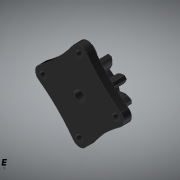
# Autodesk Inventor part: m2z10
Saved by Autodesk Inventor 2020 (Build 240168000, 168)
## iProperties
Created: 2019-05-28
Part Number: m2z10
Material: アルミニウム 2014-T4
Document SubType Name: Modeling
Designer: hamaa
Density: 2.8 g/cm^3
Appearance: サテン
Mass: 8.90635 g
Surface Area: 23.1017 cm^2
Volume: 3.18084 cm^3
Author: hamaa
Autodesk Inventor part; units mm, degrees
note: some values were not read from the file. Chosen so that the rebuilt part matches the saved one: sketch regions of "押し出し5".
ref_plane "YZ Plane" through (0, 0, 0) normal (1, 0, 0) x (0, 1, 0)
ref_plane "XZ Plane" through (0, 0, 0) normal (0, 1, 0) x (-1, 0, 0)
ref_plane "XY Plane" through (0, 0, 0) normal (0, 0, 1) x (1, 0, 0)
sketch "スケッチ1" plane through (0, 0, 0) normal (0, 0, 1) x (1, 0, 0)
  arc A0 (149.895, 114.5174) -> (149.8316, 114.302) centre (151.0075, 114.073) ccw
  arc A1 (150.3048, 115.256) -> (149.895, 114.5174) centre (153.0017, 113.2765) ccw
  arc A2 (151.645, 116.5804) -> (150.3048, 115.256) centre (155.1281, 111.7157) ccw
  arc A3 (144.0343, 113.5196) -> (144.1097, 113.3081) centre (145.1956, 113.8141) ccw
  arc A4 (143.9318, 114.3581) -> (144.0343, 113.5196) centre (147.2771, 114.3418) ccw
  arc A5 (144.2375, 116.2174) -> (143.9318, 114.3581) centre (149.9148, 114.329) ccw
  arc A6 (139.8794, 109.2677) -> (140.0647, 109.1408) centre (140.6459, 110.1884) ccw
  arc A7 (139.3036, 109.8857) -> (139.8794, 109.2677) centre (142.0196, 111.8388) ccw
  arc A8 (138.4581, 111.5696) -> (139.3036, 109.8857) centre (144.1611, 113.3789) ccw
  arc A9 (139.0173, 103.3856) -> (139.2417, 103.3918) centre (139.0961, 104.581) ccw
  arc A10 (138.1882, 103.5471) -> (139.0173, 103.3856) centre (139.2374, 106.7236) ccw
  arc A11 (136.5144, 104.4124) -> (138.1882, 103.5471) centre (140.0647, 109.2283) ccw
  arc A12 (141.7772, 98.1201) -> (141.9551, 98.2571) centre (141.1383, 99.1335) ccw
  arc A13 (141.0115, 97.7634) -> (141.7772, 98.1201) centre (139.9932, 100.95) ccw
  arc A14 (139.1487, 97.4797) -> (141.0115, 97.7634) centre (139.1903, 103.4626) ccw
  arc A15 (147.105, 95.4824) -> (147.1684, 95.6978) centre (145.9925, 95.9268) ccw
  arc A16 (146.6952, 94.7438) -> (147.105, 95.4824) centre (143.9983, 96.7233) ccw
  arc A17 (145.355, 93.4194) -> (146.6952, 94.7438) centre (141.8719, 98.2841) ccw
  arc A18 (152.9656, 96.4802) -> (152.8903, 96.6917) centre (151.8044, 96.1857) ccw
  arc A19 (153.0682, 95.6417) -> (152.9656, 96.4802) centre (149.7229, 95.658) ccw
  arc A20 (152.7625, 93.7824) -> (153.0682, 95.6417) centre (147.0852, 95.6708) ccw
  arc A21 (157.1206, 100.7321) -> (156.9353, 100.859) centre (156.3541, 99.8114) ccw
  arc A22 (157.6964, 100.1141) -> (157.1206, 100.7321) centre (154.9804, 98.161) ccw
  arc A23 (158.5419, 98.4302) -> (157.6964, 100.1141) centre (152.8389, 96.6209) ccw
  arc A24 (157.9827, 106.6143) -> (157.7583, 106.608) centre (157.9039, 105.4188) ccw
  arc A25 (158.8118, 106.4527) -> (157.9827, 106.6143) centre (157.7626, 103.2762) ccw
  arc A26 (160.4856, 105.5874) -> (158.8118, 106.4527) centre (156.9353, 100.7715) ccw
  arc A27 (155.2228, 111.8797) -> (155.0449, 111.7427) centre (155.8617, 110.8663) ccw
  arc A28 (155.9885, 112.2364) -> (155.2228, 111.8797) centre (157.0068, 109.0498) ccw
  arc A29 (157.8512, 112.5201) -> (155.9885, 112.2364) centre (157.8097, 106.5372) ccw
  arc A30 (147.1684, 114.302) -> (147.105, 114.5174) centre (145.9925, 114.073) ccw
  arc A31 (147.105, 114.5174) -> (146.6952, 115.256) centre (143.9983, 113.2765) ccw
  arc A32 (146.6952, 115.256) -> (145.355, 116.5804) centre (141.8719, 111.7157) ccw
  arc A33 (141.9551, 111.7427) -> (141.7772, 111.8797) centre (141.1383, 110.8663) ccw
  arc A34 (141.7772, 111.8797) -> (141.0115, 112.2364) centre (139.9932, 109.0498) ccw
  arc A35 (141.0115, 112.2364) -> (139.1487, 112.5201) centre (139.1903, 106.5372) ccw
  arc A36 (139.2417, 106.608) -> (139.0173, 106.6143) centre (139.0961, 105.4188) ccw
  arc A37 (139.0173, 106.6143) -> (138.1882, 106.4527) centre (139.2374, 103.2762) ccw
  arc A38 (138.1882, 106.4527) -> (136.5144, 105.5874) centre (140.0647, 100.7715) ccw
  arc A39 (140.0647, 100.859) -> (139.8794, 100.7321) centre (140.6459, 99.8114) ccw
  arc A40 (139.8794, 100.7321) -> (139.3036, 100.1141) centre (142.0196, 98.161) ccw
  arc A41 (139.3036, 100.1141) -> (138.4581, 98.4302) centre (144.1611, 96.6209) ccw
  arc A42 (144.1097, 96.6917) -> (144.0343, 96.4802) centre (145.1956, 96.1857) ccw
  arc A43 (144.0343, 96.4802) -> (143.9318, 95.6417) centre (147.2771, 95.658) ccw
  arc A44 (143.9318, 95.6417) -> (144.2375, 93.7824) centre (149.9148, 95.6708) ccw
  arc A45 (149.8316, 95.6978) -> (149.895, 95.4824) centre (151.0075, 95.9268) ccw
  arc A46 (149.895, 95.4824) -> (150.3048, 94.7438) centre (153.0017, 96.7233) ccw
  arc A47 (150.3048, 94.7438) -> (151.645, 93.4194) centre (155.1281, 98.2841) ccw
  arc A48 (155.0449, 98.2571) -> (155.2228, 98.1201) centre (155.8617, 99.1335) ccw
  arc A49 (155.2228, 98.1201) -> (155.9885, 97.7634) centre (157.0068, 100.95) ccw
  arc A50 (155.9885, 97.7634) -> (157.8512, 97.4797) centre (157.8097, 103.4626) ccw
  arc A51 (157.7583, 103.3918) -> (157.9827, 103.3856) centre (157.9039, 104.581) ccw
  arc A52 (157.9827, 103.3856) -> (158.8118, 103.5471) centre (157.7626, 106.7236) ccw
  arc A53 (158.8118, 103.5471) -> (160.4856, 104.4124) centre (156.9353, 109.2283) ccw
  arc A54 (156.9353, 109.1408) -> (157.1206, 109.2677) centre (156.3541, 110.1884) ccw
  arc A55 (157.1206, 109.2677) -> (157.6964, 109.8857) centre (154.9804, 111.8388) ccw
  arc A56 (157.6964, 109.8857) -> (158.5419, 111.5696) centre (152.8389, 113.3789) ccw
  arc A57 (152.8903, 113.3081) -> (152.9656, 113.5196) centre (151.8044, 113.8141) ccw
  arc A58 (152.9656, 113.5196) -> (153.0682, 114.3581) centre (149.7229, 114.3418) ccw
  arc A59 (153.0682, 114.3581) -> (152.7625, 116.2174) centre (147.0852, 114.329) ccw
  arc A60 (149.5628, 112.4242) -> (147.4372, 112.4242) centre (148.5, 104.9999) ccw
  arc A61 (144.9959, 111.631) -> (143.2763, 110.3816) centre (148.5, 104.9999) ccw
  arc A62 (141.7675, 108.3049) -> (141.1106, 106.2833) centre (148.5, 104.9999) ccw
  arc A63 (141.1106, 103.7165) -> (141.7675, 101.6949) centre (148.5, 104.9999) ccw
  arc A64 (143.2763, 99.6182) -> (144.9959, 98.3688) centre (148.5, 104.9999) ccw
  arc A65 (147.4372, 97.5756) -> (149.5628, 97.5756) centre (148.5, 104.9999) ccw
  arc A66 (152.0041, 98.3688) -> (153.7237, 99.6182) centre (148.5, 104.9999) ccw
  arc A67 (155.2325, 101.6949) -> (155.8894, 103.7165) centre (148.5, 104.9999) ccw
  arc A68 (155.8894, 106.2833) -> (155.2325, 108.3049) centre (148.5, 104.9999) ccw
  arc A69 (153.7237, 110.3816) -> (152.0041, 111.631) centre (148.5, 104.9999) ccw
  arc A70 (145.355, 116.5804) -> (144.2375, 116.2174) centre (148.5, 104.9999) ccw
  arc A71 (139.1487, 112.5201) -> (138.4581, 111.5696) centre (148.5, 104.9999) ccw
  arc A72 (136.5144, 105.5874) -> (136.5144, 104.4124) centre (148.5, 104.9999) ccw
  arc A73 (138.4581, 98.4302) -> (139.1487, 97.4797) centre (148.5, 104.9999) ccw
  arc A74 (144.2375, 93.7824) -> (145.355, 93.4194) centre (148.5, 104.9999) ccw
  arc A75 (151.645, 93.4194) -> (152.7625, 93.7824) centre (148.5, 104.9999) ccw
  arc A76 (157.8512, 97.4797) -> (158.5419, 98.4302) centre (148.5, 104.9999) ccw
  arc A77 (160.4856, 104.4124) -> (160.4856, 105.5874) centre (148.5, 104.9999) ccw
  arc A78 (158.5419, 111.5696) -> (157.8512, 112.5201) centre (148.5, 104.9999) ccw
  arc A79 (152.7625, 116.2174) -> (151.645, 116.5804) centre (148.5, 104.9999) ccw
  line L0 (149.5628, 112.4242) -> (149.8316, 114.302)
  line L1 (144.9959, 111.631) -> (144.1097, 113.3081)
  line L2 (141.7675, 108.3049) -> (140.0647, 109.1408)
  line L3 (141.1106, 103.7165) -> (139.2417, 103.3918)
  line L4 (143.2763, 99.6182) -> (141.9551, 98.2571)
  line L5 (147.4372, 97.5756) -> (147.1684, 95.6978)
  line L6 (152.0041, 98.3688) -> (152.8903, 96.6917)
  line L7 (155.2325, 101.6949) -> (156.9353, 100.859)
  line L8 (155.8894, 106.2833) -> (157.7583, 106.608)
  line L9 (153.7237, 110.3816) -> (155.0449, 111.7427)
  line L10 (147.4372, 112.4242) -> (147.1684, 114.302)
  line L11 (143.2763, 110.3816) -> (141.9551, 111.7427)
  line L12 (141.1106, 106.2833) -> (139.2417, 106.608)
  line L13 (141.7675, 101.6949) -> (140.0647, 100.859)
  line L14 (144.9959, 98.3688) -> (144.1097, 96.6917)
  line L15 (149.5628, 97.5756) -> (149.8316, 95.6978)
  line L16 (153.7237, 99.6182) -> (155.0449, 98.2571)
  line L17 (155.8894, 103.7165) -> (157.7583, 103.3918)
  line L18 (155.2325, 108.3049) -> (156.9353, 109.1408)
  line L19 (152.0041, 111.631) -> (152.8903, 113.3081)
  line L20 (134.5, 105) -> (162.5, 105)
  line L21 (148.5, 91) -> (148.5, 119)
  line L22 (180.5, 116.9999) -> (250.5, 116.9999)
  line L23 (180.5, 108.9999) -> (250.5, 108.9999)
  line L24 (180.5, 100.9999) -> (250.5, 100.9999)
  line L25 (180.5, 92.9999) -> (250.5, 92.9999)
  line L26 (180.5, 84.9999) -> (250.5, 84.9999)
  line L27 (180.5, 76.9999) -> (250.5, 76.9999)
  line L28 (180.5, 68.9999) -> (250.5, 68.9999)
  line L29 (180.5, 60.9999) -> (250.5, 60.9999)
  line L30 (180.5, 52.9999) -> (250.5, 52.9999)
  line L31 (180.5, 44.9999) -> (250.5, 44.9999)
  line L32 (180.5, 36.9999) -> (250.5, 36.9999)
  line L33 (180.5, 28.9999) -> (250.5, 28.9999)
  line L34 (180.5, 20.9999) -> (250.5, 20.9999)
  line L35 (180.5, 116.9999) -> (180.5, 20.9999)
  line L36 (250.5, 116.9999) -> (250.5, 20.9999)
  line L37 (215.5, 108.9999) -> (215.5, 20.9999)
  point P0 (0, 0)
  point P1 (186.5, 111)
  point P2 (189, 103)
  point P3 (189, 95)
  point P4 (186.5, 87)
  point P5 (189, 79)
  point P6 (184, 71)
  point P7 (186.5, 63)
  point P8 (186.5, 55)
  point P9 (186.5, 47)
  point P10 (189, 39)
  point P11 (189, 31)
  point P12 (186.5, 23)
  point P13 (216.5, 103)
  point P14 (231.5, 95)
  point P15 (232.75, 87)
  point P16 (229, 79)
  point P17 (231.5, 71)
  point P18 (225.25, 63)
  point P19 (231.5, 55)
  point P20 (231.5, 47)
  point P21 (226.5, 39)
  point P22 (234, 31)
  point P23 (234, 23)
  point P24 (149.5, 132.5)
  point P25 (149.5, 126.5)
  point P26 (166.75, 132.5)
  point P27 (167.8125, 126.5)
  constraints: 160 point on circle, 80 centre point, 72 end point, 60 tangent, 57 equal radius, 23 parallel, 2 horizontal, 2 midpoint, 2 perpendicular, 55 other
extrude "押し出し1" add sketch "スケッチ1" along normal blind 5 contours A1 A2 A79 A59 A58 A57 L19 A69 L9 A27 A28 A29 A78 A56 A55 A54 L18 A68 L8 A24 A25 A26 A77 L20 L21 A60 L0 A0 | L21 L20 A72 A38 A37 A36 L12 A62 L2 A6 A7 A8 A71 A35 A34 A33 L11 A61 L1 A3 A4 A5 A70 A32 A31 A30 L10 A60 | L21 A65 L5 A15 A16 A17 A74 A44 A43 A42 L14 A64 L4 A12 A13 A14 A73 A41 A40 A39 L13 A63 L3 A9 A10 A11 A72 L20 | L20 A77 A53 A52 A51 L17 A67 L7 A21 A22 A23 A76 A50 A49 A48 L16 A66 L6 A18 A19 A20 A75 A47 A46 A45 L15 A65 L21
sketch "スケッチ2" plane through (0, 0, 5) normal (0, 0, 1) x (1, 0, 0)
  arc A0 (149.895, 114.5174) -> (149.8316, 114.302) centre (151.0075, 114.073) ccw projected
  line L0 (149.8316, 114.302) -> (149.5628, 112.4242) projected
  arc A1 (149.5628, 112.4242) -> (147.4372, 112.4242) centre (148.5, 104.9999) ccw projected
  line L1 (147.4372, 112.4242) -> (147.1684, 114.302) projected
  arc A2 (147.1684, 114.302) -> (147.105, 114.5174) centre (145.9925, 114.073) ccw projected
  arc A3 (147.105, 114.5174) -> (146.6952, 115.256) centre (143.9983, 113.2765) ccw projected
  arc A4 (146.6952, 115.256) -> (145.355, 116.5804) centre (141.8719, 111.7157) ccw projected
  arc A5 (145.355, 116.5804) -> (144.2375, 116.2174) centre (148.5, 104.9999) ccw projected
  arc A6 (144.2375, 116.2174) -> (143.9318, 114.3581) centre (149.9148, 114.329) ccw projected
  arc A7 (143.9318, 114.3581) -> (144.0343, 113.5196) centre (147.2771, 114.3418) ccw projected
  arc A8 (144.0343, 113.5196) -> (144.1097, 113.3081) centre (145.1956, 113.8141) ccw projected
  line L2 (144.1097, 113.3081) -> (144.9959, 111.631) projected
  arc A9 (144.9959, 111.631) -> (143.2763, 110.3816) centre (148.5, 104.9999) ccw projected
  line L3 (143.2763, 110.3816) -> (141.9551, 111.7427) projected
  arc A10 (141.9551, 111.7427) -> (141.7772, 111.8797) centre (141.1383, 110.8663) ccw projected
  arc A11 (141.7772, 111.8797) -> (141.0115, 112.2364) centre (139.9932, 109.0498) ccw projected
  arc A12 (141.0115, 112.2364) -> (139.1487, 112.5201) centre (139.1903, 106.5372) ccw projected
  arc A13 (139.1487, 112.5201) -> (138.4581, 111.5696) centre (148.5, 104.9999) ccw projected
  arc A14 (138.4581, 111.5696) -> (139.3036, 109.8857) centre (144.1611, 113.3789) ccw projected
  arc A15 (139.3036, 109.8857) -> (139.8794, 109.2677) centre (142.0196, 111.8388) ccw projected
  arc A16 (139.8794, 109.2677) -> (140.0647, 109.1408) centre (140.6459, 110.1884) ccw projected
  line L4 (140.0647, 109.1408) -> (141.7675, 108.3049) projected
  arc A17 (141.7675, 108.3049) -> (141.1106, 106.2833) centre (148.5, 104.9999) ccw projected
  line L5 (141.1106, 106.2833) -> (139.2417, 106.608) projected
  arc A18 (139.2417, 106.608) -> (139.0173, 106.6143) centre (139.0961, 105.4188) ccw projected
  arc A19 (139.0173, 106.6143) -> (138.1882, 106.4527) centre (139.2374, 103.2762) ccw projected
  arc A20 (138.1882, 106.4527) -> (136.5144, 105.5874) centre (140.0647, 100.7715) ccw projected
  arc A21 (136.5144, 105.5874) -> (136.5144, 104.4124) centre (148.5, 104.9999) ccw projected
  arc A22 (136.5144, 104.4124) -> (138.1882, 103.5471) centre (140.0647, 109.2283) ccw projected
  arc A23 (138.1882, 103.5471) -> (139.0173, 103.3856) centre (139.2374, 106.7236) ccw projected
  arc A24 (139.0173, 103.3856) -> (139.2417, 103.3918) centre (139.0961, 104.581) ccw projected
  line L6 (139.2417, 103.3918) -> (141.1106, 103.7165) projected
  arc A25 (141.1106, 103.7165) -> (141.7675, 101.6949) centre (148.5, 104.9999) ccw projected
  line L7 (141.7675, 101.6949) -> (140.0647, 100.859) projected
  arc A26 (140.0647, 100.859) -> (139.8794, 100.7321) centre (140.6459, 99.8114) ccw projected
  arc A27 (139.8794, 100.7321) -> (139.3036, 100.1141) centre (142.0196, 98.161) ccw projected
  arc A28 (139.3036, 100.1141) -> (138.4581, 98.4302) centre (144.1611, 96.6209) ccw projected
  arc A29 (138.4581, 98.4302) -> (139.1487, 97.4797) centre (148.5, 104.9999) ccw projected
  arc A30 (139.1487, 97.4797) -> (141.0115, 97.7634) centre (139.1903, 103.4626) ccw projected
  arc A31 (141.0115, 97.7634) -> (141.7772, 98.1201) centre (139.9932, 100.95) ccw projected
  arc A32 (141.7772, 98.1201) -> (141.9551, 98.2571) centre (141.1383, 99.1335) ccw projected
  line L8 (141.9551, 98.2571) -> (143.2763, 99.6182) projected
  arc A33 (143.2763, 99.6182) -> (144.9959, 98.3688) centre (148.5, 104.9999) ccw projected
  line L9 (144.9959, 98.3688) -> (144.1097, 96.6917) projected
  arc A34 (144.1097, 96.6917) -> (144.0343, 96.4802) centre (145.1956, 96.1857) ccw projected
  arc A35 (144.0343, 96.4802) -> (143.9318, 95.6417) centre (147.2771, 95.658) ccw projected
  arc A36 (143.9318, 95.6417) -> (144.2375, 93.7824) centre (149.9148, 95.6708) ccw projected
  arc A37 (144.2375, 93.7824) -> (145.355, 93.4194) centre (148.5, 104.9999) ccw projected
  arc A38 (145.355, 93.4194) -> (146.6952, 94.7438) centre (141.8719, 98.2841) ccw projected
  arc A39 (146.6952, 94.7438) -> (147.105, 95.4824) centre (143.9983, 96.7233) ccw projected
  arc A40 (147.105, 95.4824) -> (147.1684, 95.6978) centre (145.9925, 95.9268) ccw projected
  line L10 (147.1684, 95.6978) -> (147.4372, 97.5756) projected
  arc A41 (147.4372, 97.5756) -> (149.5628, 97.5756) centre (148.5, 104.9999) ccw projected
  line L11 (149.5628, 97.5756) -> (149.8316, 95.6978) projected
  arc A42 (149.8316, 95.6978) -> (149.895, 95.4824) centre (151.0075, 95.9268) ccw projected
  arc A43 (149.895, 95.4824) -> (150.3048, 94.7438) centre (153.0017, 96.7233) ccw projected
  arc A44 (150.3048, 94.7438) -> (151.645, 93.4194) centre (155.1281, 98.2841) ccw projected
  arc A45 (151.645, 93.4194) -> (152.7625, 93.7824) centre (148.5, 104.9999) ccw projected
  arc A46 (152.7625, 93.7824) -> (153.0682, 95.6417) centre (147.0852, 95.6708) ccw projected
  arc A47 (153.0682, 95.6417) -> (152.9656, 96.4802) centre (149.7229, 95.658) ccw projected
  arc A48 (152.9656, 96.4802) -> (152.8903, 96.6917) centre (151.8044, 96.1857) ccw projected
  line L12 (152.8903, 96.6917) -> (152.0041, 98.3688) projected
  arc A49 (152.0041, 98.3688) -> (153.7237, 99.6182) centre (148.5, 104.9999) ccw projected
  line L13 (153.7237, 99.6182) -> (155.0449, 98.2571) projected
  arc A50 (155.0449, 98.2571) -> (155.2228, 98.1201) centre (155.8617, 99.1335) ccw projected
  arc A51 (155.2228, 98.1201) -> (155.9885, 97.7634) centre (157.0068, 100.95) ccw projected
  arc A52 (155.9885, 97.7634) -> (157.8512, 97.4797) centre (157.8097, 103.4626) ccw projected
  arc A53 (157.8512, 97.4797) -> (158.5419, 98.4302) centre (148.5, 104.9999) ccw projected
  arc A54 (158.5419, 98.4302) -> (157.6964, 100.1141) centre (152.8389, 96.6209) ccw projected
  arc A55 (157.6964, 100.1141) -> (157.1206, 100.7321) centre (154.9804, 98.161) ccw projected
  arc A56 (157.1206, 100.7321) -> (156.9353, 100.859) centre (156.3541, 99.8114) ccw projected
  line L14 (156.9353, 100.859) -> (155.2325, 101.6949) projected
  arc A57 (155.2325, 101.6949) -> (155.8894, 103.7165) centre (148.5, 104.9999) ccw projected
  line L15 (155.8894, 103.7165) -> (157.7583, 103.3918) projected
  arc A58 (157.7583, 103.3918) -> (157.9827, 103.3856) centre (157.9039, 104.581) ccw projected
  arc A59 (157.9827, 103.3856) -> (158.8118, 103.5471) centre (157.7626, 106.7236) ccw projected
  arc A60 (158.8118, 103.5471) -> (160.4856, 104.4124) centre (156.9353, 109.2283) ccw projected
  arc A61 (160.4856, 104.4124) -> (160.4856, 105.5874) centre (148.5, 104.9999) ccw projected
  arc A62 (160.4856, 105.5874) -> (158.8118, 106.4527) centre (156.9353, 100.7715) ccw projected
  arc A63 (158.8118, 106.4527) -> (157.9827, 106.6143) centre (157.7626, 103.2762) ccw projected
  arc A64 (157.9827, 106.6143) -> (157.7583, 106.608) centre (157.9039, 105.4188) ccw projected
  line L16 (157.7583, 106.608) -> (155.8894, 106.2833) projected
  arc A65 (155.8894, 106.2833) -> (155.2325, 108.3049) centre (148.5, 104.9999) ccw projected
  line L17 (155.2325, 108.3049) -> (156.9353, 109.1408) projected
  arc A66 (156.9353, 109.1408) -> (157.1206, 109.2677) centre (156.3541, 110.1884) ccw projected
  arc A67 (157.1206, 109.2677) -> (157.6964, 109.8857) centre (154.9804, 111.8388) ccw projected
  arc A68 (157.6964, 109.8857) -> (158.5419, 111.5696) centre (152.8389, 113.3789) ccw projected
  arc A69 (158.5419, 111.5696) -> (157.8512, 112.5201) centre (148.5, 104.9999) ccw projected
  arc A70 (157.8512, 112.5201) -> (155.9885, 112.2364) centre (157.8097, 106.5372) ccw projected
  arc A71 (155.9885, 112.2364) -> (155.2228, 111.8797) centre (157.0068, 109.0498) ccw projected
  arc A72 (155.2228, 111.8797) -> (155.0449, 111.7427) centre (155.8617, 110.8663) ccw projected
  line L18 (155.0449, 111.7427) -> (153.7237, 110.3816) projected
  arc A73 (153.7237, 110.3816) -> (152.0041, 111.631) centre (148.5, 104.9999) ccw projected
  line L19 (152.0041, 111.631) -> (152.8903, 113.3081) projected
  arc A74 (152.8903, 113.3081) -> (152.9656, 113.5196) centre (151.8044, 113.8141) ccw projected
  arc A75 (152.9656, 113.5196) -> (153.0682, 114.3581) centre (149.7229, 114.3418) ccw projected
  arc A76 (153.0682, 114.3581) -> (152.7625, 116.2174) centre (147.0852, 114.329) ccw projected
  arc A77 (152.7625, 116.2174) -> (151.645, 116.5804) centre (148.5, 104.9999) ccw projected
  arc A78 (151.645, 116.5804) -> (150.3048, 115.256) centre (155.1281, 111.7157) ccw projected
  arc A79 (150.3048, 115.256) -> (149.895, 114.5174) centre (153.0017, 113.2765) ccw projected
  circle A80 centre (148.5, 104.9999) radius 5
  circle A81 centre (148.5, 104.9999) radius 5.6
  point P0 (0, 0)
  dimension "d2" = 10
  dimension "d3" = 0.6
  constraints: 2 centre point, 1 coincident
  measures "d2" diameter of A80
  measures "d3" radial gap between concentric circles of A80 A81
extrude "押し出し2" cut sketch "スケッチ2" against normal blind 10 contours A80
extrude "押し出し3" cut sketch "スケッチ2" against normal blind 0.6 contours A81
sketch "スケッチ3" plane through (0, 0, 5) normal (0, 0, 1) x (1, 0, 0)
  arc A0 (142.9838, 117.9197) -> (135.5802, 110.5161) centre (148.5, 104.9999) ccw
  arc A1 (144.308, 117.3636) -> (142.9838, 117.9197) centre (143.3765, 117) ccw
  arc A2 (144.308, 117.3636) -> (152.692, 117.3636) centre (148.5, 118.9999) ccw
  arc A3 (154.0162, 117.9197) -> (152.692, 117.3636) centre (153.6235, 117) ccw
  arc A4 (161.4198, 110.5161) -> (154.0162, 117.9197) centre (148.5, 104.9999) ccw
  arc A5 (160.8637, 109.1919) -> (161.4198, 110.5161) centre (160.5001, 110.1234) ccw
  arc A6 (160.8637, 109.1919) -> (160.8637, 100.8079) centre (162.5, 104.9999) ccw
  arc A7 (161.4198, 99.4837) -> (160.8637, 100.8079) centre (160.5001, 99.8764) ccw
  arc A8 (154.0162, 92.0801) -> (161.4198, 99.4837) centre (148.5, 104.9999) ccw
  arc A9 (152.692, 92.6362) -> (154.0162, 92.0801) centre (153.6235, 92.9998) ccw
  arc A10 (152.692, 92.6362) -> (144.308, 92.6362) centre (148.5, 90.9999) ccw
  arc A11 (142.9838, 92.0801) -> (144.308, 92.6362) centre (143.3765, 92.9998) ccw
  arc A12 (135.5802, 99.4837) -> (142.9838, 92.0801) centre (148.5, 104.9999) ccw
  arc A13 (136.1362, 100.8079) -> (135.5802, 99.4837) centre (136.4999, 99.8764) ccw
  arc A14 (136.1362, 100.8079) -> (136.1362, 109.1919) centre (134.5, 104.9999) ccw
  arc A15 (135.5802, 110.5161) -> (136.1362, 109.1919) centre (136.4999, 110.1234) ccw
  circle A16 centre (162.5, 104.9999) radius 1.5
  circle A17 centre (134.5, 104.9999) radius 1.5
  circle A18 centre (148.5, 90.9999) radius 1.5
  circle A19 centre (148.5, 118.9999) radius 1.5
  circle A20 centre (148.5, 104.9999) radius 18.25
  circle A21 centre (148.5, 104.9999) radius 5.6 projected
  arc A22 (149.895, 114.5174) -> (149.8316, 114.302) centre (151.0075, 114.073) ccw projected
  line L0 (149.8316, 114.302) -> (149.5628, 112.4242) projected
  arc A23 (149.5628, 112.4242) -> (147.4372, 112.4242) centre (148.5, 104.9999) ccw projected
  line L1 (147.4372, 112.4242) -> (147.1684, 114.302) projected
  arc A24 (147.1684, 114.302) -> (147.105, 114.5174) centre (145.9925, 114.073) ccw projected
  arc A25 (147.105, 114.5174) -> (146.6952, 115.256) centre (143.9983, 113.2765) ccw projected
  arc A26 (146.6952, 115.256) -> (145.355, 116.5804) centre (141.8719, 111.7157) ccw projected
  arc A27 (145.355, 116.5804) -> (144.2375, 116.2174) centre (148.5, 104.9999) ccw projected
  arc A28 (144.2375, 116.2174) -> (143.9318, 114.3581) centre (149.9148, 114.329) ccw projected
  arc A29 (143.9318, 114.3581) -> (144.0343, 113.5196) centre (147.2771, 114.3418) ccw projected
  arc A30 (144.0343, 113.5196) -> (144.1097, 113.3081) centre (145.1956, 113.8141) ccw projected
  line L2 (144.1097, 113.3081) -> (144.9959, 111.631) projected
  arc A31 (144.9959, 111.631) -> (143.2763, 110.3816) centre (148.5, 104.9999) ccw projected
  line L3 (143.2763, 110.3816) -> (141.9551, 111.7427) projected
  arc A32 (141.9551, 111.7427) -> (141.7772, 111.8797) centre (141.1383, 110.8663) ccw projected
  arc A33 (141.7772, 111.8797) -> (141.0115, 112.2364) centre (139.9932, 109.0498) ccw projected
  arc A34 (141.0115, 112.2364) -> (139.1487, 112.5201) centre (139.1903, 106.5372) ccw projected
  arc A35 (139.1487, 112.5201) -> (138.4581, 111.5696) centre (148.5, 104.9999) ccw projected
  arc A36 (138.4581, 111.5696) -> (139.3036, 109.8857) centre (144.1611, 113.3789) ccw projected
  arc A37 (139.3036, 109.8857) -> (139.8794, 109.2677) centre (142.0196, 111.8388) ccw projected
  arc A38 (139.8794, 109.2677) -> (140.0647, 109.1408) centre (140.6459, 110.1884) ccw projected
  line L4 (140.0647, 109.1408) -> (141.7675, 108.3049) projected
  arc A39 (141.7675, 108.3049) -> (141.1106, 106.2833) centre (148.5, 104.9999) ccw projected
  line L5 (141.1106, 106.2833) -> (139.2417, 106.608) projected
  arc A40 (139.2417, 106.608) -> (139.0173, 106.6143) centre (139.0961, 105.4188) ccw projected
  arc A41 (139.0173, 106.6143) -> (138.1882, 106.4527) centre (139.2374, 103.2762) ccw projected
  arc A42 (138.1882, 106.4527) -> (136.5144, 105.5874) centre (140.0647, 100.7715) ccw projected
  arc A43 (136.5144, 105.5874) -> (136.5144, 104.4124) centre (148.5, 104.9999) ccw projected
  arc A44 (136.5144, 104.4124) -> (138.1882, 103.5471) centre (140.0647, 109.2283) ccw projected
  arc A45 (138.1882, 103.5471) -> (139.0173, 103.3856) centre (139.2374, 106.7236) ccw projected
  arc A46 (139.0173, 103.3856) -> (139.2417, 103.3918) centre (139.0961, 104.581) ccw projected
  line L6 (139.2417, 103.3918) -> (141.1106, 103.7165) projected
  arc A47 (141.1106, 103.7165) -> (141.7675, 101.6949) centre (148.5, 104.9999) ccw projected
  line L7 (141.7675, 101.6949) -> (140.0647, 100.859) projected
  arc A48 (140.0647, 100.859) -> (139.8794, 100.7321) centre (140.6459, 99.8114) ccw projected
  arc A49 (139.8794, 100.7321) -> (139.3036, 100.1141) centre (142.0196, 98.161) ccw projected
  arc A50 (139.3036, 100.1141) -> (138.4581, 98.4302) centre (144.1611, 96.6209) ccw projected
  arc A51 (138.4581, 98.4302) -> (139.1487, 97.4797) centre (148.5, 104.9999) ccw projected
  arc A52 (139.1487, 97.4797) -> (141.0115, 97.7634) centre (139.1903, 103.4626) ccw projected
  arc A53 (141.0115, 97.7634) -> (141.7772, 98.1201) centre (139.9932, 100.95) ccw projected
  arc A54 (141.7772, 98.1201) -> (141.9551, 98.2571) centre (141.1383, 99.1335) ccw projected
  line L8 (141.9551, 98.2571) -> (143.2763, 99.6182) projected
  arc A55 (143.2763, 99.6182) -> (144.9959, 98.3688) centre (148.5, 104.9999) ccw projected
  line L9 (144.9959, 98.3688) -> (144.1097, 96.6917) projected
  arc A56 (144.1097, 96.6917) -> (144.0343, 96.4802) centre (145.1956, 96.1857) ccw projected
  arc A57 (144.0343, 96.4802) -> (143.9318, 95.6417) centre (147.2771, 95.658) ccw projected
  arc A58 (143.9318, 95.6417) -> (144.2375, 93.7824) centre (149.9148, 95.6708) ccw projected
  arc A59 (144.2375, 93.7824) -> (145.355, 93.4194) centre (148.5, 104.9999) ccw projected
  arc A60 (145.355, 93.4194) -> (146.6952, 94.7438) centre (141.8719, 98.2841) ccw projected
  arc A61 (146.6952, 94.7438) -> (147.105, 95.4824) centre (143.9983, 96.7233) ccw projected
  arc A62 (147.105, 95.4824) -> (147.1684, 95.6978) centre (145.9925, 95.9268) ccw projected
  line L10 (147.1684, 95.6978) -> (147.4372, 97.5756) projected
  arc A63 (147.4372, 97.5756) -> (149.5628, 97.5756) centre (148.5, 104.9999) ccw projected
  line L11 (149.5628, 97.5756) -> (149.8316, 95.6978) projected
  arc A64 (149.8316, 95.6978) -> (149.895, 95.4824) centre (151.0075, 95.9268) ccw projected
  arc A65 (149.895, 95.4824) -> (150.3048, 94.7438) centre (153.0017, 96.7233) ccw projected
  arc A66 (150.3048, 94.7438) -> (151.645, 93.4194) centre (155.1281, 98.2841) ccw projected
  arc A67 (151.645, 93.4194) -> (152.7625, 93.7824) centre (148.5, 104.9999) ccw projected
  arc A68 (152.7625, 93.7824) -> (153.0682, 95.6417) centre (147.0852, 95.6708) ccw projected
  arc A69 (153.0682, 95.6417) -> (152.9656, 96.4802) centre (149.7229, 95.658) ccw projected
  arc A70 (152.9656, 96.4802) -> (152.8903, 96.6917) centre (151.8044, 96.1857) ccw projected
  line L12 (152.8903, 96.6917) -> (152.0041, 98.3688) projected
  arc A71 (152.0041, 98.3688) -> (153.7237, 99.6182) centre (148.5, 104.9999) ccw projected
  line L13 (153.7237, 99.6182) -> (155.0449, 98.2571) projected
  arc A72 (155.0449, 98.2571) -> (155.2228, 98.1201) centre (155.8617, 99.1335) ccw projected
  arc A73 (155.2228, 98.1201) -> (155.9885, 97.7634) centre (157.0068, 100.95) ccw projected
  arc A74 (155.9885, 97.7634) -> (157.8512, 97.4797) centre (157.8097, 103.4626) ccw projected
  arc A75 (157.8512, 97.4797) -> (158.5419, 98.4302) centre (148.5, 104.9999) ccw projected
  arc A76 (158.5419, 98.4302) -> (157.6964, 100.1141) centre (152.8389, 96.6209) ccw projected
  arc A77 (157.6964, 100.1141) -> (157.1206, 100.7321) centre (154.9804, 98.161) ccw projected
  arc A78 (157.1206, 100.7321) -> (156.9353, 100.859) centre (156.3541, 99.8114) ccw projected
  line L14 (156.9353, 100.859) -> (155.2325, 101.6949) projected
  arc A79 (155.2325, 101.6949) -> (155.8894, 103.7165) centre (148.5, 104.9999) ccw projected
  line L15 (155.8894, 103.7165) -> (157.7583, 103.3918) projected
  arc A80 (157.7583, 103.3918) -> (157.9827, 103.3856) centre (157.9039, 104.581) ccw projected
  arc A81 (157.9827, 103.3856) -> (158.8118, 103.5471) centre (157.7626, 106.7236) ccw projected
  arc A82 (158.8118, 103.5471) -> (160.4856, 104.4124) centre (156.9353, 109.2283) ccw projected
  arc A83 (160.4856, 104.4124) -> (160.4856, 105.5874) centre (148.5, 104.9999) ccw projected
  arc A84 (160.4856, 105.5874) -> (158.8118, 106.4527) centre (156.9353, 100.7715) ccw projected
  arc A85 (158.8118, 106.4527) -> (157.9827, 106.6143) centre (157.7626, 103.2762) ccw projected
  arc A86 (157.9827, 106.6143) -> (157.7583, 106.608) centre (157.9039, 105.4188) ccw projected
  line L16 (157.7583, 106.608) -> (155.8894, 106.2833) projected
  arc A87 (155.8894, 106.2833) -> (155.2325, 108.3049) centre (148.5, 104.9999) ccw projected
  line L17 (155.2325, 108.3049) -> (156.9353, 109.1408) projected
  arc A88 (156.9353, 109.1408) -> (157.1206, 109.2677) centre (156.3541, 110.1884) ccw projected
  arc A89 (157.1206, 109.2677) -> (157.6964, 109.8857) centre (154.9804, 111.8388) ccw projected
  arc A90 (157.6964, 109.8857) -> (158.5419, 111.5696) centre (152.8389, 113.3789) ccw projected
  arc A91 (158.5419, 111.5696) -> (157.8512, 112.5201) centre (148.5, 104.9999) ccw projected
  arc A92 (157.8512, 112.5201) -> (155.9885, 112.2364) centre (157.8097, 106.5372) ccw projected
  arc A93 (155.9885, 112.2364) -> (155.2228, 111.8797) centre (157.0068, 109.0498) ccw projected
  arc A94 (155.2228, 111.8797) -> (155.0449, 111.7427) centre (155.8617, 110.8663) ccw projected
  line L18 (155.0449, 111.7427) -> (153.7237, 110.3816) projected
  arc A95 (153.7237, 110.3816) -> (152.0041, 111.631) centre (148.5, 104.9999) ccw projected
  line L19 (152.0041, 111.631) -> (152.8903, 113.3081) projected
  arc A96 (152.8903, 113.3081) -> (152.9656, 113.5196) centre (151.8044, 113.8141) ccw projected
  arc A97 (152.9656, 113.5196) -> (153.0682, 114.3581) centre (149.7229, 114.3418) ccw projected
  arc A98 (153.0682, 114.3581) -> (152.7625, 116.2174) centre (147.0852, 114.329) ccw projected
  arc A99 (152.7625, 116.2174) -> (151.645, 116.5804) centre (148.5, 104.9999) ccw projected
  arc A100 (151.645, 116.5804) -> (150.3048, 115.256) centre (155.1281, 111.7157) ccw projected
  arc A101 (150.3048, 115.256) -> (149.895, 114.5174) centre (153.0017, 113.2765) ccw projected
  point P0 (0, 0)
  constraints: 32 point on circle, 21 centre point
sketch "スケッチ4" plane through (0, 0, 5) normal (0, 0, 1) x (1, 0, 0)
  circle A0 centre (148.5, 118.9999) radius 1.5 construction
  circle A1 centre (134.5, 104.9999) radius 1.5 construction
  circle A2 centre (162.5, 104.9999) radius 1.5 construction
  circle A3 centre (148.5, 90.9999) radius 1.5 construction
  circle A4 centre (148.5, 104.9999) radius 5.6 projected
  arc A5 (149.895, 114.5174) -> (149.8316, 114.302) centre (151.0075, 114.073) ccw projected
  line L0 (149.8316, 114.302) -> (149.5628, 112.4242) projected
  arc A6 (149.5628, 112.4242) -> (147.4372, 112.4242) centre (148.5, 104.9999) ccw projected
  line L1 (147.4372, 112.4242) -> (147.1684, 114.302) projected
  arc A7 (147.1684, 114.302) -> (147.105, 114.5174) centre (145.9925, 114.073) ccw projected
  arc A8 (147.105, 114.5174) -> (146.6952, 115.256) centre (143.9983, 113.2765) ccw projected
  arc A9 (146.6952, 115.256) -> (145.355, 116.5804) centre (141.8719, 111.7157) ccw projected
  arc A10 (145.355, 116.5804) -> (144.2375, 116.2174) centre (148.5, 104.9999) ccw projected
  arc A11 (144.2375, 116.2174) -> (143.9318, 114.3581) centre (149.9148, 114.329) ccw projected
  arc A12 (143.9318, 114.3581) -> (144.0343, 113.5196) centre (147.2771, 114.3418) ccw projected
  arc A13 (144.0343, 113.5196) -> (144.1097, 113.3081) centre (145.1956, 113.8141) ccw projected
  line L2 (144.1097, 113.3081) -> (144.9959, 111.631) projected
  arc A14 (144.9959, 111.631) -> (143.2763, 110.3816) centre (148.5, 104.9999) ccw projected
  line L3 (143.2763, 110.3816) -> (141.9551, 111.7427) projected
  arc A15 (141.9551, 111.7427) -> (141.7772, 111.8797) centre (141.1383, 110.8663) ccw projected
  arc A16 (141.7772, 111.8797) -> (141.0115, 112.2364) centre (139.9932, 109.0498) ccw projected
  arc A17 (141.0115, 112.2364) -> (139.1487, 112.5201) centre (139.1903, 106.5372) ccw projected
  arc A18 (139.1487, 112.5201) -> (138.4581, 111.5696) centre (148.5, 104.9999) ccw projected
  arc A19 (138.4581, 111.5696) -> (139.3036, 109.8857) centre (144.1611, 113.3789) ccw projected
  arc A20 (139.3036, 109.8857) -> (139.8794, 109.2677) centre (142.0196, 111.8388) ccw projected
  arc A21 (139.8794, 109.2677) -> (140.0647, 109.1408) centre (140.6459, 110.1884) ccw projected
  line L4 (140.0647, 109.1408) -> (141.7675, 108.3049) projected
  arc A22 (141.7675, 108.3049) -> (141.1106, 106.2833) centre (148.5, 104.9999) ccw projected
  line L5 (141.1106, 106.2833) -> (139.2417, 106.608) projected
  arc A23 (139.2417, 106.608) -> (139.0173, 106.6143) centre (139.0961, 105.4188) ccw projected
  arc A24 (139.0173, 106.6143) -> (138.1882, 106.4527) centre (139.2374, 103.2762) ccw projected
  arc A25 (138.1882, 106.4527) -> (136.5144, 105.5874) centre (140.0647, 100.7715) ccw projected
  arc A26 (136.5144, 105.5874) -> (136.5144, 104.4124) centre (148.5, 104.9999) ccw projected
  arc A27 (136.5144, 104.4124) -> (138.1882, 103.5471) centre (140.0647, 109.2283) ccw projected
  arc A28 (138.1882, 103.5471) -> (139.0173, 103.3856) centre (139.2374, 106.7236) ccw projected
  arc A29 (139.0173, 103.3856) -> (139.2417, 103.3918) centre (139.0961, 104.581) ccw projected
  line L6 (139.2417, 103.3918) -> (141.1106, 103.7165) projected
  arc A30 (141.1106, 103.7165) -> (141.7675, 101.6949) centre (148.5, 104.9999) ccw projected
  line L7 (141.7675, 101.6949) -> (140.0647, 100.859) projected
  arc A31 (140.0647, 100.859) -> (139.8794, 100.7321) centre (140.6459, 99.8114) ccw projected
  arc A32 (139.8794, 100.7321) -> (139.3036, 100.1141) centre (142.0196, 98.161) ccw projected
  arc A33 (139.3036, 100.1141) -> (138.4581, 98.4302) centre (144.1611, 96.6209) ccw projected
  arc A34 (138.4581, 98.4302) -> (139.1487, 97.4797) centre (148.5, 104.9999) ccw projected
  arc A35 (139.1487, 97.4797) -> (141.0115, 97.7634) centre (139.1903, 103.4626) ccw projected
  arc A36 (141.0115, 97.7634) -> (141.7772, 98.1201) centre (139.9932, 100.95) ccw projected
  arc A37 (141.7772, 98.1201) -> (141.9551, 98.2571) centre (141.1383, 99.1335) ccw projected
  line L8 (141.9551, 98.2571) -> (143.2763, 99.6182) projected
  arc A38 (143.2763, 99.6182) -> (144.9959, 98.3688) centre (148.5, 104.9999) ccw projected
  line L9 (144.9959, 98.3688) -> (144.1097, 96.6917) projected
  arc A39 (144.1097, 96.6917) -> (144.0343, 96.4802) centre (145.1956, 96.1857) ccw projected
  arc A40 (144.0343, 96.4802) -> (143.9318, 95.6417) centre (147.2771, 95.658) ccw projected
  arc A41 (143.9318, 95.6417) -> (144.2375, 93.7824) centre (149.9148, 95.6708) ccw projected
  arc A42 (144.2375, 93.7824) -> (145.355, 93.4194) centre (148.5, 104.9999) ccw projected
  arc A43 (145.355, 93.4194) -> (146.6952, 94.7438) centre (141.8719, 98.2841) ccw projected
  arc A44 (146.6952, 94.7438) -> (147.105, 95.4824) centre (143.9983, 96.7233) ccw projected
  arc A45 (147.105, 95.4824) -> (147.1684, 95.6978) centre (145.9925, 95.9268) ccw projected
  line L10 (147.1684, 95.6978) -> (147.4372, 97.5756) projected
  arc A46 (147.4372, 97.5756) -> (149.5628, 97.5756) centre (148.5, 104.9999) ccw projected
  line L11 (149.5628, 97.5756) -> (149.8316, 95.6978) projected
  arc A47 (149.8316, 95.6978) -> (149.895, 95.4824) centre (151.0075, 95.9268) ccw projected
  arc A48 (149.895, 95.4824) -> (150.3048, 94.7438) centre (153.0017, 96.7233) ccw projected
  arc A49 (150.3048, 94.7438) -> (151.645, 93.4194) centre (155.1281, 98.2841) ccw projected
  arc A50 (151.645, 93.4194) -> (152.7625, 93.7824) centre (148.5, 104.9999) ccw projected
  arc A51 (152.7625, 93.7824) -> (153.0682, 95.6417) centre (147.0852, 95.6708) ccw projected
  arc A52 (153.0682, 95.6417) -> (152.9656, 96.4802) centre (149.7229, 95.658) ccw projected
  arc A53 (152.9656, 96.4802) -> (152.8903, 96.6917) centre (151.8044, 96.1857) ccw projected
  line L12 (152.8903, 96.6917) -> (152.0041, 98.3688) projected
  arc A54 (152.0041, 98.3688) -> (153.7237, 99.6182) centre (148.5, 104.9999) ccw projected
  line L13 (153.7237, 99.6182) -> (155.0449, 98.2571) projected
  arc A55 (155.0449, 98.2571) -> (155.2228, 98.1201) centre (155.8617, 99.1335) ccw projected
  arc A56 (155.2228, 98.1201) -> (155.9885, 97.7634) centre (157.0068, 100.95) ccw projected
  arc A57 (155.9885, 97.7634) -> (157.8512, 97.4797) centre (157.8097, 103.4626) ccw projected
  arc A58 (157.8512, 97.4797) -> (158.5419, 98.4302) centre (148.5, 104.9999) ccw projected
  arc A59 (158.5419, 98.4302) -> (157.6964, 100.1141) centre (152.8389, 96.6209) ccw projected
  arc A60 (157.6964, 100.1141) -> (157.1206, 100.7321) centre (154.9804, 98.161) ccw projected
  arc A61 (157.1206, 100.7321) -> (156.9353, 100.859) centre (156.3541, 99.8114) ccw projected
  line L14 (156.9353, 100.859) -> (155.2325, 101.6949) projected
  arc A62 (155.2325, 101.6949) -> (155.8894, 103.7165) centre (148.5, 104.9999) ccw projected
  line L15 (155.8894, 103.7165) -> (157.7583, 103.3918) projected
  arc A63 (157.7583, 103.3918) -> (157.9827, 103.3856) centre (157.9039, 104.581) ccw projected
  arc A64 (157.9827, 103.3856) -> (158.8118, 103.5471) centre (157.7626, 106.7236) ccw projected
  arc A65 (158.8118, 103.5471) -> (160.4856, 104.4124) centre (156.9353, 109.2283) ccw projected
  arc A66 (160.4856, 104.4124) -> (160.4856, 105.5874) centre (148.5, 104.9999) ccw projected
  arc A67 (160.4856, 105.5874) -> (158.8118, 106.4527) centre (156.9353, 100.7715) ccw projected
  arc A68 (158.8118, 106.4527) -> (157.9827, 106.6143) centre (157.7626, 103.2762) ccw projected
  arc A69 (157.9827, 106.6143) -> (157.7583, 106.608) centre (157.9039, 105.4188) ccw projected
  line L16 (157.7583, 106.608) -> (155.8894, 106.2833) projected
  arc A70 (155.8894, 106.2833) -> (155.2325, 108.3049) centre (148.5, 104.9999) ccw projected
  line L17 (155.2325, 108.3049) -> (156.9353, 109.1408) projected
  arc A71 (156.9353, 109.1408) -> (157.1206, 109.2677) centre (156.3541, 110.1884) ccw projected
  arc A72 (157.1206, 109.2677) -> (157.6964, 109.8857) centre (154.9804, 111.8388) ccw projected
  arc A73 (157.6964, 109.8857) -> (158.5419, 111.5696) centre (152.8389, 113.3789) ccw projected
  arc A74 (158.5419, 111.5696) -> (157.8512, 112.5201) centre (148.5, 104.9999) ccw projected
  arc A75 (157.8512, 112.5201) -> (155.9885, 112.2364) centre (157.8097, 106.5372) ccw projected
  arc A76 (155.9885, 112.2364) -> (155.2228, 111.8797) centre (157.0068, 109.0498) ccw projected
  arc A77 (155.2228, 111.8797) -> (155.0449, 111.7427) centre (155.8617, 110.8663) ccw projected
  line L18 (155.0449, 111.7427) -> (153.7237, 110.3816) projected
  arc A78 (153.7237, 110.3816) -> (152.0041, 111.631) centre (148.5, 104.9999) ccw projected
  line L19 (152.0041, 111.631) -> (152.8903, 113.3081) projected
  arc A79 (152.8903, 113.3081) -> (152.9656, 113.5196) centre (151.8044, 113.8141) ccw projected
  arc A80 (152.9656, 113.5196) -> (153.0682, 114.3581) centre (149.7229, 114.3418) ccw projected
  arc A81 (153.0682, 114.3581) -> (152.7625, 116.2174) centre (147.0852, 114.329) ccw projected
  arc A82 (152.7625, 116.2174) -> (151.645, 116.5804) centre (148.5, 104.9999) ccw projected
  arc A83 (151.645, 116.5804) -> (150.3048, 115.256) centre (155.1281, 111.7157) ccw projected
  arc A84 (150.3048, 115.256) -> (149.895, 114.5174) centre (153.0017, 113.2765) ccw projected
  circle A85 centre (148.5, 118.9999) radius 1.25
  circle A86 centre (162.5, 104.9999) radius 1.25
  circle A87 centre (148.5, 90.9999) radius 1.25
  circle A88 centre (134.5, 104.9999) radius 1.25
  circle A89 centre (148.5, 104.9999) radius 1.995
  circle A90 centre (148.5, 118.9999) radius 3
  circle A91 centre (134.5, 104.9999) radius 3
  circle A92 centre (148.5, 90.9999) radius 3
  circle A93 centre (162.5, 104.9999) radius 3
  circle A94 centre (148.5, 104.9999) radius 12.1
  arc A95 (150.9342, 120.7533) -> (164.2534, 107.4341) centre (198.555, 155.0549) ccw
  arc A96 (164.2534, 102.5657) -> (150.9342, 89.2465) centre (198.555, 54.9449) ccw
  arc A97 (146.0657, 89.2465) -> (132.7466, 102.5657) centre (98.445, 54.9449) ccw
  arc A98 (132.7466, 107.4341) -> (146.0657, 120.7533) centre (98.445, 155.0549) ccw
  point P0 (0, 0)
  dimension "d8" = 2.5
  dimension "d9" = 2.5
  dimension "d10" = 2.5
  dimension "d11" = 2.5
  dimension "d12" = 3.99
  dimension "d13" = 6
  dimension "d14" = 6
  dimension "d15" = 6
  dimension "d16" = 6
  dimension "d17" = 0.1
  constraints: 16 point on circle, 14 centre point, 12 tangent, 10 coincident
  measures "d8" diameter of A85
  measures "d9" diameter of A86
  measures "d10" diameter of A87
  measures "d11" diameter of A88
  measures "d12" diameter of A89
  measures "d13" diameter of A90
  measures "d14" diameter of A91
  measures "d15" diameter of A92
  measures "d16" diameter of A93
  measures "d17" radial gap between concentric circles of A74 A94
extrude "押し出し4" add sketch "スケッチ4" against normal blind 5 contours A4
extrude "押し出し5" add sketch "スケッチ4" along normal blind 3 contours A4 | A84 A83 A82 A81 A80 A79 L19 A78 L18 A77 A76 A75 A74 A73 A72 A71 L17 A70 L16 A69 A68 A67 A93 A65 A64 A63 L15 A62 L14 A61 A60 A59 A58 A57 A56 A55 L13 A54 L12 A53 A52 A51 A50 A49 A48 A47 L11 A46 L10 A45 A44 A43 A42 A41 A40 A39 L9 A38 L8 A37 A36 A35 A34 A33 A32 A31 L7 A30 L6 A29 A28 A27 A91 A25 A24 A23 L5 A22 L4 A21 A20 A19 A18 A17 A16 A15 L3 A14 L2 A13 A12 A11 A10 A9 A8 A7 L1 A6 L0 A5 | A5 L0 A6 L1 A7 A8 A9 A10 A11 A12 A13 L2 A14 L3 A15 A16 A17 A18 A19 A20 A21 L4 A22 L5 A23 A24 A25 A91 A94 A90 A93 A67 A68 A69 L16 A70 L17 A71 A72 A73 A74 A75 A76 A77 L18 A78 L19 A79 A80 A81 A82 A83 A84 | A93 A94 A65 A66 A67 | A67 A66 A65 A93 | A94 A95 A93 | A93 A94 | A93 A94 A92 A91 A27 A28 A29 L6 A30 L7 A31 A32 A33 A34 A35 A36 A37 L8 A38 L9 A39 A40 A41 A42 A43 A44 A45 L10 A46 L11 A47 A48 A49 A50 A51 A52 A53 L12 A54 L13 A55 A56 A57 A58 A59 A60 A61 L14 A62 L15 A63 A64 A65 | A94 A90 A95 | A93 A96 A94 | A94 A90 | A90 A94 | A96 A92 A94 | A94 A98 A90 | A94 A92 | A92 A94 | A91 A27 A26 A25 | A25 A26 A27 A91 A94 | A94 A91 A98 | A92 A97 A94 | A94 A91 | A97 A91 A94
sketch "スケッチ5" plane through (0, 0, 0) normal (0, 0, -1) x (-1, 0, 0)
  circle A0 centre (-148.5, 104.9999) radius 1.995 projected
  arc A1 (-149.8316, 114.302) -> (-149.895, 114.5174) centre (-151.0075, 114.073) ccw projected
  arc A2 (-149.895, 114.5174) -> (-150.3048, 115.256) centre (-153.0017, 113.2765) ccw projected
  arc A3 (-150.3048, 115.256) -> (-151.645, 116.5804) centre (-155.1281, 111.7157) ccw projected
  arc A4 (-151.645, 116.5804) -> (-152.7625, 116.2174) centre (-148.5, 104.9999) ccw projected
  arc A5 (-152.7625, 116.2174) -> (-153.0682, 114.3581) centre (-147.0852, 114.329) ccw projected
  arc A6 (-153.0682, 114.3581) -> (-152.9656, 113.5196) centre (-149.7229, 114.3418) ccw projected
  arc A7 (-152.9656, 113.5196) -> (-152.8903, 113.3081) centre (-151.8044, 113.8141) ccw projected
  line L0 (-152.0041, 111.631) -> (-152.8903, 113.3081) projected
  arc A8 (-152.0041, 111.631) -> (-153.7237, 110.3816) centre (-148.5, 104.9999) ccw projected
  line L1 (-155.0449, 111.7427) -> (-153.7237, 110.3816) projected
  arc A9 (-155.0449, 111.7427) -> (-155.2228, 111.8797) centre (-155.8617, 110.8663) ccw projected
  arc A10 (-155.2228, 111.8797) -> (-155.9885, 112.2364) centre (-157.0068, 109.0498) ccw projected
  arc A11 (-155.9885, 112.2364) -> (-157.8512, 112.5201) centre (-157.8097, 106.5372) ccw projected
  arc A12 (-157.8512, 112.5201) -> (-158.5419, 111.5696) centre (-148.5, 104.9999) ccw projected
  arc A13 (-158.5419, 111.5696) -> (-157.6964, 109.8857) centre (-152.8389, 113.3789) ccw projected
  arc A14 (-157.6964, 109.8857) -> (-157.1206, 109.2677) centre (-154.9804, 111.8388) ccw projected
  arc A15 (-157.1206, 109.2677) -> (-156.9353, 109.1408) centre (-156.3541, 110.1884) ccw projected
  line L2 (-155.2325, 108.3049) -> (-156.9353, 109.1408) projected
  arc A16 (-155.2325, 108.3049) -> (-155.8894, 106.2833) centre (-148.5, 104.9999) ccw projected
  line L3 (-157.7583, 106.608) -> (-155.8894, 106.2833) projected
  arc A17 (-157.7583, 106.608) -> (-157.9827, 106.6143) centre (-157.9039, 105.4188) ccw projected
  arc A18 (-157.9827, 106.6143) -> (-158.8118, 106.4527) centre (-157.7626, 103.2762) ccw projected
  arc A19 (-158.8118, 106.4527) -> (-160.4856, 105.5874) centre (-156.9353, 100.7715) ccw projected
  arc A20 (-160.4856, 105.5874) -> (-160.4856, 104.4124) centre (-148.5, 104.9999) ccw projected
  arc A21 (-160.4856, 104.4124) -> (-158.8118, 103.5471) centre (-156.9353, 109.2283) ccw projected
  arc A22 (-158.8118, 103.5471) -> (-157.9827, 103.3856) centre (-157.7626, 106.7236) ccw projected
  arc A23 (-157.9827, 103.3856) -> (-157.7583, 103.3918) centre (-157.9039, 104.581) ccw projected
  line L4 (-155.8894, 103.7165) -> (-157.7583, 103.3918) projected
  arc A24 (-155.8894, 103.7165) -> (-155.2325, 101.6949) centre (-148.5, 104.9999) ccw projected
  line L5 (-156.9353, 100.859) -> (-155.2325, 101.6949) projected
  arc A25 (-156.9353, 100.859) -> (-157.1206, 100.7321) centre (-156.3541, 99.8114) ccw projected
  arc A26 (-157.1206, 100.7321) -> (-157.6964, 100.1141) centre (-154.9804, 98.161) ccw projected
  arc A27 (-157.6964, 100.1141) -> (-158.5419, 98.4302) centre (-152.8389, 96.6209) ccw projected
  arc A28 (-158.5419, 98.4302) -> (-157.8512, 97.4797) centre (-148.5, 104.9999) ccw projected
  arc A29 (-157.8512, 97.4797) -> (-155.9885, 97.7634) centre (-157.8097, 103.4626) ccw projected
  arc A30 (-155.9885, 97.7634) -> (-155.2228, 98.1201) centre (-157.0068, 100.95) ccw projected
  arc A31 (-155.2228, 98.1201) -> (-155.0449, 98.2571) centre (-155.8617, 99.1335) ccw projected
  line L6 (-153.7237, 99.6182) -> (-155.0449, 98.2571) projected
  arc A32 (-153.7237, 99.6182) -> (-152.0041, 98.3688) centre (-148.5, 104.9999) ccw projected
  line L7 (-152.8903, 96.6917) -> (-152.0041, 98.3688) projected
  arc A33 (-152.8903, 96.6917) -> (-152.9656, 96.4802) centre (-151.8044, 96.1857) ccw projected
  arc A34 (-152.9656, 96.4802) -> (-153.0682, 95.6417) centre (-149.7229, 95.658) ccw projected
  arc A35 (-153.0682, 95.6417) -> (-152.7625, 93.7824) centre (-147.0852, 95.6708) ccw projected
  arc A36 (-152.7625, 93.7824) -> (-151.645, 93.4194) centre (-148.5, 104.9999) ccw projected
  arc A37 (-151.645, 93.4194) -> (-150.3048, 94.7438) centre (-155.1281, 98.2841) ccw projected
  arc A38 (-150.3048, 94.7438) -> (-149.895, 95.4824) centre (-153.0017, 96.7233) ccw projected
  arc A39 (-149.895, 95.4824) -> (-149.8316, 95.6978) centre (-151.0075, 95.9268) ccw projected
  line L8 (-149.5628, 97.5756) -> (-149.8316, 95.6978) projected
  arc A40 (-149.5628, 97.5756) -> (-147.4372, 97.5756) centre (-148.5, 104.9999) ccw projected
  line L9 (-147.1684, 95.6978) -> (-147.4372, 97.5756) projected
  arc A41 (-147.1684, 95.6978) -> (-147.105, 95.4824) centre (-145.9925, 95.9268) ccw projected
  arc A42 (-147.105, 95.4824) -> (-146.6952, 94.7438) centre (-143.9983, 96.7233) ccw projected
  arc A43 (-146.6952, 94.7438) -> (-145.355, 93.4194) centre (-141.8719, 98.2841) ccw projected
  arc A44 (-145.355, 93.4194) -> (-144.2375, 93.7824) centre (-148.5, 104.9999) ccw projected
  arc A45 (-144.2375, 93.7824) -> (-143.9318, 95.6417) centre (-149.9148, 95.6708) ccw projected
  arc A46 (-143.9318, 95.6417) -> (-144.0343, 96.4802) centre (-147.2771, 95.658) ccw projected
  arc A47 (-144.0343, 96.4802) -> (-144.1097, 96.6917) centre (-145.1956, 96.1857) ccw projected
  line L10 (-144.9959, 98.3688) -> (-144.1097, 96.6917) projected
  arc A48 (-144.9959, 98.3688) -> (-143.2763, 99.6182) centre (-148.5, 104.9999) ccw projected
  line L11 (-141.9551, 98.2571) -> (-143.2763, 99.6182) projected
  arc A49 (-141.9551, 98.2571) -> (-141.7772, 98.1201) centre (-141.1383, 99.1335) ccw projected
  arc A50 (-141.7772, 98.1201) -> (-141.0115, 97.7634) centre (-139.9932, 100.95) ccw projected
  arc A51 (-141.0115, 97.7634) -> (-139.1487, 97.4797) centre (-139.1903, 103.4626) ccw projected
  arc A52 (-139.1487, 97.4797) -> (-138.4581, 98.4302) centre (-148.5, 104.9999) ccw projected
  arc A53 (-138.4581, 98.4302) -> (-139.3036, 100.1141) centre (-144.1611, 96.6209) ccw projected
  arc A54 (-139.3036, 100.1141) -> (-139.8794, 100.7321) centre (-142.0196, 98.161) ccw projected
  arc A55 (-139.8794, 100.7321) -> (-140.0647, 100.859) centre (-140.6459, 99.8114) ccw projected
  line L12 (-141.7675, 101.6949) -> (-140.0647, 100.859) projected
  arc A56 (-141.7675, 101.6949) -> (-141.1106, 103.7165) centre (-148.5, 104.9999) ccw projected
  line L13 (-139.2417, 103.3918) -> (-141.1106, 103.7165) projected
  arc A57 (-139.2417, 103.3918) -> (-139.0173, 103.3856) centre (-139.0961, 104.581) ccw projected
  arc A58 (-139.0173, 103.3856) -> (-138.1882, 103.5471) centre (-139.2374, 106.7236) ccw projected
  arc A59 (-138.1882, 103.5471) -> (-136.5144, 104.4124) centre (-140.0647, 109.2283) ccw projected
  arc A60 (-136.5144, 104.4124) -> (-136.5144, 105.5874) centre (-148.5, 104.9999) ccw projected
  arc A61 (-136.5144, 105.5874) -> (-138.1882, 106.4527) centre (-140.0647, 100.7715) ccw projected
  arc A62 (-138.1882, 106.4527) -> (-139.0173, 106.6143) centre (-139.2374, 103.2762) ccw projected
  arc A63 (-139.0173, 106.6143) -> (-139.2417, 106.608) centre (-139.0961, 105.4188) ccw projected
  line L14 (-141.1106, 106.2833) -> (-139.2417, 106.608) projected
  arc A64 (-141.1106, 106.2833) -> (-141.7675, 108.3049) centre (-148.5, 104.9999) ccw projected
  line L15 (-140.0647, 109.1408) -> (-141.7675, 108.3049) projected
  arc A65 (-140.0647, 109.1408) -> (-139.8794, 109.2677) centre (-140.6459, 110.1884) ccw projected
  arc A66 (-139.8794, 109.2677) -> (-139.3036, 109.8857) centre (-142.0196, 111.8388) ccw projected
  arc A67 (-139.3036, 109.8857) -> (-138.4581, 111.5696) centre (-144.1611, 113.3789) ccw projected
  arc A68 (-138.4581, 111.5696) -> (-139.1487, 112.5201) centre (-148.5, 104.9999) ccw projected
  arc A69 (-139.1487, 112.5201) -> (-141.0115, 112.2364) centre (-139.1903, 106.5372) ccw projected
  arc A70 (-141.0115, 112.2364) -> (-141.7772, 111.8797) centre (-139.9932, 109.0498) ccw projected
  arc A71 (-141.7772, 111.8797) -> (-141.9551, 111.7427) centre (-141.1383, 110.8663) ccw projected
  line L16 (-143.2763, 110.3816) -> (-141.9551, 111.7427) projected
  arc A72 (-143.2763, 110.3816) -> (-144.9959, 111.631) centre (-148.5, 104.9999) ccw projected
  line L17 (-144.1097, 113.3081) -> (-144.9959, 111.631) projected
  arc A73 (-144.1097, 113.3081) -> (-144.0343, 113.5196) centre (-145.1956, 113.8141) ccw projected
  arc A74 (-144.0343, 113.5196) -> (-143.9318, 114.3581) centre (-147.2771, 114.3418) ccw projected
  arc A75 (-143.9318, 114.3581) -> (-144.2375, 116.2174) centre (-149.9148, 114.329) ccw projected
  arc A76 (-144.2375, 116.2174) -> (-145.355, 116.5804) centre (-148.5, 104.9999) ccw projected
  arc A77 (-145.355, 116.5804) -> (-146.6952, 115.256) centre (-141.8719, 111.7157) ccw projected
  arc A78 (-146.6952, 115.256) -> (-147.105, 114.5174) centre (-143.9983, 113.2765) ccw projected
  arc A79 (-147.105, 114.5174) -> (-147.1684, 114.302) centre (-145.9925, 114.073) ccw projected
  line L18 (-147.4372, 112.4242) -> (-147.1684, 114.302) projected
  arc A80 (-147.4372, 112.4242) -> (-149.5628, 112.4242) centre (-148.5, 104.9999) ccw projected
  line L19 (-149.8316, 114.302) -> (-149.5628, 112.4242) projected
  circle A81 centre (-162.5, 104.9999) radius 1.25 projected
  circle A82 centre (-148.5, 90.9999) radius 1.25 projected
  circle A83 centre (-134.5, 104.9999) radius 1.25 projected
  circle A84 centre (-148.5, 118.9999) radius 1.25 projected
  arc A85 (-146.0657, 120.7533) -> (-132.7466, 107.4341) centre (-98.445, 155.0549) ccw projected
  arc A86 (-132.7466, 102.5657) -> (-132.7466, 107.4341) centre (-134.5, 104.9999) ccw projected
  arc A87 (-132.7466, 102.5657) -> (-146.0657, 89.2465) centre (-98.445, 54.9449) ccw projected
  arc A88 (-150.9342, 89.2465) -> (-146.0657, 89.2465) centre (-148.5, 90.9999) ccw projected
  arc A89 (-150.9342, 89.2465) -> (-164.2534, 102.5657) centre (-198.555, 54.9449) ccw projected
  arc A90 (-164.2534, 107.4341) -> (-164.2534, 102.5657) centre (-162.5, 104.9999) ccw projected
  arc A91 (-164.2534, 107.4341) -> (-150.9342, 120.7533) centre (-198.555, 155.0549) ccw projected
  arc A92 (-146.0657, 120.7533) -> (-150.9342, 120.7533) centre (-148.5, 118.9999) ccw projected
  circle A93 centre (-148.5, 104.9999) radius 1.995 projected
  circle A94 centre (-148.5, 104.9999) radius 12
  point P0 (0, 0)
  constraints: 1 coincident, 3 other
